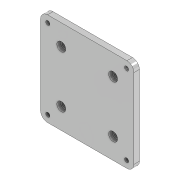
# Autodesk Inventor part: plaat aan stoel
Saved by Autodesk Inventor 2020.3 (Build 243373000, 373)
## iProperties
Created: 2020-09-16
Part Number: plaat aan stoel
Material: Aluminum 6061
Document SubType Name: Modeling
Designer: Svend
Density: 2.7 g/cm^3
Appearance: Aluminum - Polished
Author: Svend
Autodesk Inventor part; units mm, degrees
ref_plane "YZ Plane" through (0, 0, 0) normal (1, 0, 0) x (0, 1, 0)
ref_plane "XZ Plane" through (0, 0, 0) normal (0, 1, 0) x (-1, 0, 0)
ref_plane "XY Plane" through (0, 0, 0) normal (0, 0, 1) x (1, 0, 0)
sketch "Sketch1" plane through (0, 0, 0) normal (0, 0, 1) x (1, 0, 0)
  circle A0 centre (-57, 57.5) radius 3
  circle A1 centre (57, 57.5) radius 3
  circle A2 centre (-57, -57.5) radius 3
  circle A3 centre (57, -57.5) radius 3
  line L0 (-57, 57.5) -> (57, -57.5) construction
  line L1 (-57, -57.5) -> (57, 57.5) construction
  line L2 (-67.5, 67.5) -> (67.5, 67.5)
  line L3 (67.5, 67.5) -> (67.5, -67.5)
  line L4 (67.5, -67.5) -> (-67.5, -67.5)
  line L5 (-67.5, -67.5) -> (-67.5, 67.5)
  line L6 (-67.5, 67.5) -> (67.5, -67.5) construction
  line L7 (67.5, 67.5) -> (-67.5, -67.5) construction
  circle A4 centre (-37.5, 37.5) radius 4
  circle A5 centre (-37.5, -37.5) radius 4
  circle A6 centre (37.5, -37.5) radius 4
  circle A7 centre (37.5, 37.5) radius 4
  point P0 (0, 0)
  point P1 (0, 0)
  dimension "d0" = 114
  dimension "d1" = 115
  dimension "d2" = 6
  dimension "d3" = 135
  dimension "d4" = 135
  dimension "d5" = 8
  dimension "d6" = 30
  dimension "d9" = 360
  constraints: 16 end point, 8 centre point, 3 equal radius, 3 midpoint, 2 horizontal alignment, 2 parallel, 2 vertical alignment, 1 coincident, 1 horizontal, 1 perpendicular, 1 point on line, 9 other
  measures "d0" distance of L1.end L0.start
  measures "d1" distance of L0.end L1.end
  measures "d2" diameter of A1
  measures "d3" distance of L3.end L4.end
  measures "d4" distance of L2.end L3.end
  measures "d5" diameter of A4
  measures "d6" distance from line of L5 A4.centre
extrude "Extrusion1" add sketch "Sketch1" along normal blind 8
sketch "Sketch2" plane through (0, 0, 8) normal (0, 0, 1) x (1, 0, 0)
  line L0 (-67.5, -67.5) -> (67.5, -67.5) projected
  line L1 (67.5, -67.5) -> (67.5, 67.5) projected
  line L2 (67.5, 67.5) -> (-67.5, 67.5) projected
  line L3 (-67.5, 67.5) -> (-67.5, -67.5) projected
  circle A0 centre (37.5, 37.5) radius 4 projected
  circle A1 centre (37.5, -37.5) radius 4 projected
  circle A2 centre (-37.5, -37.5) radius 4 projected
  circle A3 centre (-37.5, 37.5) radius 4 projected
  circle A4 centre (57, -57.5) radius 3 projected
  circle A5 centre (-57, -57.5) radius 3 projected
  circle A6 centre (57, 57.5) radius 3 projected
  circle A7 centre (-57, 57.5) radius 3 projected
  circle A8 centre (-37.5, 37.5) radius 6.5
  circle A9 centre (-37.5, -37.5) radius 6.5
  circle A10 centre (37.5, -37.5) radius 6.5
  circle A11 centre (37.5, 37.5) radius 6.5
  point P0 (0, 0)
  dimension "d13" = 13
  dimension "d16" = 360
  constraints: 4 centre point, 1 coincident, 9 other
  measures "d13" diameter of A8
extrude "Extrusion2" cut sketch "Sketch2" against normal blind 5 contours A0 | A1 | A2 | A3 | A8 | A9 | A10 | A11
fillet "Fillet1" radius 10 4 edges at (-67.5, 67.5, 4) (67.5, 67.5, 4) (-67.5, -67.5, 4) (67.5, -67.5, 4)
thread "Thread1" size "M6x1" class "6H" standard "ANSI Metric M Profile" full length
thread "Thread2" size "M6x1" class "6H" standard "ANSI Metric M Profile" full length
thread "Thread3" size "M6x1" class "6H" standard "ANSI Metric M Profile" full length
thread "Thread4" size "M6x1" class "6H" standard "ANSI Metric M Profile" full length
body "Solid1"
